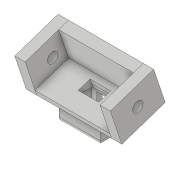
# Autodesk Inventor part: Lidar Sensor Case v2
Saved by Autodesk Inventor 2018.3 (Build 223284000, 284)
## iProperties
Created: 2019-02-04
Part Number: Lidar Sensor Case v2
Material: Generic
Document SubType Name: Modeling
Designer: aye06091
Mass: 21.1942 g
Surface Area: 105.081 cm^2
Volume: 21.1942 cm^3
Density: 1 g/cm^3
Appearance: Default
Author: aye06091
Autodesk Inventor part; units mm, degrees
ref_plane "YZ Plane" through (0, 0, 0) normal (1, 0, 0) x (0, 1, 0)
ref_plane "XZ Plane" through (0, 0, 0) normal (0, 1, 0) x (-1, 0, 0)
ref_plane "XY Plane" through (0, 0, 0) normal (0, 0, 1) x (1, 0, 0)
sketch "Sketch8" plane through (0, 0, 0) normal (1, 0, 0) x (0, 1, 0)
  line L0 (-3.8078, 7.851) -> (3.0591, -12.6251)
  line L1 (-0.2897, -12.6251) -> (-4.6863, 0.485)
  line L2 (3.0591, -12.6251) -> (-0.2897, -12.6251)
  line L3 (-4.6863, 0.485) -> (-6.818, 6.8414)
  line L4 (-3.8078, 7.851) -> (-6.818, 6.8414)
  point P0 (0, 0)
  constraints: 10 end point, 1 horizontal, 1 perpendicular
extrude "Extrusion6" add sketch "Sketch8" along normal blind 45.72
sketch "Sketch11" plane through (0, 0, 0) normal (-1, 0, 0) x (0, 0, 1)
  line L0 (0.485, -4.6863) -> (-12.6251, -0.2897) projected
  line L1 (7.851, -6.8159) -> (0.485, -6.8159) projected
  line L2 (7.851, -6.8159) -> (0.485, -6.8159)
  line L3 (0.485, -6.8159) -> (0.485, -4.6863)
  line L4 (-12.6251, -0.2897) -> (0.485, -4.6863)
  line L5 (7.851, -3.8078) -> (-12.6251, 3.0591) projected
  line L6 (0.485, -6.8159) -> (7.851, -6.8159) projected
  line L7 (13.9082, 14.2533) -> (7.851, -3.808)
  line L8 (7.851, -3.808) -> (-18.639, 5.076)
  line L9 (-18.639, 5.076) -> (-12.5817, 23.1373)
  line L10 (-12.5817, 23.1373) -> (13.9082, 14.2533)
  point P0 (0, 0)
  dimension "d73" = 27.94
  dimension "d74" = 18.54
  dimension "d76" = 0
  dimension "d88" = 19.05
  constraints: 14 end point, 2 parallel, 2 perpendicular, 1 point on line
  measures "d73" distance of L9.end L7.start
  measures "d74" angle of L6 L8
  measures "d76" distance from line of L5 L8.end
  measures "d88" distance of L8.end L9.end
extrude "Extrusion8" add sketch "Sketch11" along normal blind 6.35
sketch "Sketch13" plane through (0, -3.8078, 7.851) normal (0, 0.9481042, 0.3179598) x (1, 0, 0)
  line L0 (0, 0) -> (0, 21.5968) projected
  line L1 (16.51, 18.0408) -> (29.21, 18.0408)
  line L2 (29.21, 18.0408) -> (29.21, 10.4208)
  line L3 (29.21, 10.4208) -> (16.51, 10.4208)
  line L4 (16.51, 10.4208) -> (16.51, 18.0408)
  point P0 (0, 8.6543)
  dimension "d55" = 7.62
  dimension "d56" = 12.7
  dimension "d57" = 16.51
  constraints: 8 end point, 2 parallel, 1 horizontal, 1 perpendicular
  measures "d55" distance of L3.end L1.start
  measures "d56" distance of L2.end L3.end
  measures "d57" distance between parallel lines of L0 L4
extrude "Extrusion10" cut sketch "Sketch13" against normal blind 25.4
sketch "Sketch15" plane through (0, 0, 0) normal (1, 0, 0) x (0, 0, -1)
  line L0 (-0.485, -6.8159) -> (-7.851, -6.8159) projected
  line L1 (6.5678, 21.1205) -> (12.5883, 23.1395)
  line L2 (12.5883, 23.1395) -> (18.6455, 5.0782)
  line L3 (18.6455, 5.0782) -> (12.6251, 3.0591)
  line L4 (12.6251, 3.0591) -> (6.5678, 21.1205)
  dimension "d67" = 6.35
  dimension "d68" = 18.54
  dimension "d69" = 0
  dimension "d70" = 0
  dimension "d87" = 19.05
  constraints: 8 end point, 2 parallel, 1 perpendicular
  measures "d67" distance of L1.start L1.end
  measures "d68" angle of L0 L3
  measures "d69" distance of point (12.625, 3.059) L3.end
  measures "d70" distance of point (12.625, 3.059) L3.end
  measures "d87" distance of L3.end L1.start
extrude "Extrusion11" add sketch "Sketch15" along normal blind 45.72
sketch "Sketch17" plane through (45.72, 0, 0) normal (1, 0, 0) x (0, 0, -1)
  line L0 (-7.851, -3.808) -> (-13.9082, 14.2533) projected
  line L1 (-7.851, -3.808) -> (-13.9082, 14.2533)
  line L2 (-13.9082, 14.2533) -> (12.5883, 23.1395)
  line L3 (12.5883, 23.1395) -> (18.6456, 5.0782)
  line L4 (18.6456, 5.0782) -> (-7.851, -3.808)
  point P0 (0, 0)
  constraints: 8 end point, 2 parallel, 1 perpendicular
extrude "Extrusion12" add sketch "Sketch17" along normal blind 6.35
sketch "Sketch19" plane through (45.72, 5.0782, -18.6456) normal (0, -0.9481019, -0.3179666) x (1, 0, 0)
  line L0 (0, 6.3501) -> (0, 0.0001) projected
  line L1 (6.35, 27.947) -> (0, 27.947)
  line L2 (0, 27.947) -> (0, 0.0001)
  line L3 (0, 0.0001) -> (6.35, 0.0001)
  line L4 (6.35, 0.0001) -> (6.35, 27.947)
  line L5 (-45.72, 6.3501) -> (0, 6.3501) projected
  line L6 (0, 0.0001) -> (0, 0.0001)
  line L7 (0, 0.0001) -> (0, 6.3501)
  line L8 (0, 6.3501) -> (0, 6.3501)
  line L9 (0, 6.3501) -> (0, 0.0001)
  line L10 (-45.72, 0.007) -> (-52.07, 0.007) projected
  line L11 (-52.07, 0.007) -> (-45.72, 0.007)
  line L12 (-45.72, 0.007) -> (-45.72, 27.947)
  line L13 (-45.72, 27.947) -> (-52.07, 27.947)
  line L14 (-52.07, 27.947) -> (-52.07, 0.007)
  point P0 (-45.72, 19.2926)
  constraints: 24 end point, 6 equal length, 3 horizontal, 3 perpendicular, 1 point on line
extrude "Extrusion13" add sketch "Sketch19" along normal blind 3.175
sketch "Sketch20" plane through (0, 5.0782, -18.6455) normal (0, -0.9481019, -0.3179666) x (1, 0, 0)
  line L0 (45.72, 0) -> (0, 0)
  line L1 (0, 0) -> (0, 6.35)
  line L2 (0, 6.35) -> (45.72, 6.35)
  line L3 (45.72, 6.35) -> (45.72, 0)
  point P0 (0, 19.2926)
  constraints: 8 end point, 2 parallel, 1 horizontal, 1 perpendicular
extrude "Extrusion14" add sketch "Sketch20" along normal blind 3.175
sketch "Sketch21" plane through (0, 0, 0) normal (1, 0, 0) x (0, 0, -1)
  line L0 (19.6485, 2.0658) -> (13.6346, 0.0489) projected
  line L1 (13.6346, 0.0489) -> (12.6251, 3.0591) projected
  line L2 (12.6251, 3.0591) -> (12.6251, -0.2897) projected
  line L3 (12.6251, -0.2897) -> (-6.8414, -6.818) projected
  line L4 (-0.485, -4.6863) -> (-0.485, -4.6865) projected
  line L5 (19.6485, 2.0657) -> (-6.8414, -6.8182) projected
  line L6 (19.6485, 2.0657) -> (19.6485, 2.0658) projected
  line L7 (12.6251, 3.0591) -> (13.6346, 0.0489)
  line L8 (12.6251, -0.2897) -> (13.6346, 0.0489)
  line L9 (12.6251, 3.0591) -> (12.6251, -0.2897)
  point P0 (0, 0)
  point P1 (-6.8415, -6.8181)
  constraints: 6 end point, 2 collinear, 1 perpendicular
extrude "Extrusion15" add sketch "Sketch21" along normal blind 45.72
sketch "Sketch22" plane through (16.51, -1.0818, -10.2631) normal (0, 0.9481042, 0.3179598) x (1, 0, 0)
  line L0 (12.7, -7.62) -> (12.7, 0) projected
  line L1 (12.7, 0) -> (0, 0) projected
  line L2 (0, 0) -> (12.7, 0)
  line L3 (12.7, 0) -> (12.7, -7.62)
  line L4 (12.7, -7.62) -> (0, -7.62)
  line L5 (0, -7.62) -> (0, 0)
  point P0 (-16.51, -9.3866)
  constraints: 8 end point, 2 parallel, 1 horizontal, 1 perpendicular
extrude "Extrusion16" cut sketch "Sketch22" against normal blind 45.72
sketch "Sketch23" plane through (52.07, 0, 0) normal (1, 0, 0) x (0, 0, -1)
  circle A0 centre (2.8734, 8.1606) radius 3.175
  point P0 (0, 0)
  dimension "d89" = 6.35
  constraints: 1 centre point
  measures "d89" diameter of A0
extrude "Extrusion17" cut sketch "Sketch23" against normal blind 76.2
ref_plane "Work Plane1" through (0, -6.818, 6.8414) normal (0, -1, 0) x (1, 0, 0)
sketch "Sketch25" plane through (0, -6.818, 6.8414) normal (0, -1, 0) x (1, 0, 0)
  line L0 (35.56, -20.2796) -> (35.56, -3.5301)
  line L1 (35.56, -3.5301) -> (32.385, -3.5301)
  line L2 (32.385, -3.5301) -> (32.385, -20.2796)
  line L3 (32.385, -6.7051) -> (10.16, -6.7051)
  line L4 (10.16, -6.7051) -> (10.16, -3.5301)
  line L5 (10.16, -3.5301) -> (32.385, -3.5301)
  line L6 (32.385, -3.5301) -> (32.385, -6.7051)
  line L7 (10.16, -6.7051) -> (13.335, -6.7051)
  line L8 (13.335, -6.7051) -> (13.335, -20.2796)
  line L9 (10.16, -20.2796) -> (10.16, -6.7051)
  line L10 (13.335, -20.2796) -> (32.385, -20.2796)
  line L11 (32.385, -20.2796) -> (32.385, -23.4546)
  line L12 (32.385, -23.4546) -> (13.335, -23.4546)
  line L13 (13.335, -23.4546) -> (13.335, -20.2796)
  line L14 (29.21, -17.1046) -> (16.51, -17.1046) projected
  line L15 (29.21, -9.8801) -> (29.21, -17.1046) projected
  line L16 (16.51, -9.8801) -> (29.21, -9.8801) projected
  line L17 (16.51, -17.1046) -> (16.51, -9.8801) projected
  line L18 (32.385, -23.4546) -> (35.56, -23.4546)
  line L19 (35.56, -23.4546) -> (35.56, -3.5301)
  line L20 (35.56, -3.5301) -> (32.385, -3.5301)
  line L21 (32.385, -3.5301) -> (32.385, -23.4546)
  line L22 (32.385, -3.5301) -> (10.16, -3.5301)
  line L23 (10.16, -3.5301) -> (10.16, -6.7051)
  line L24 (10.16, -6.7051) -> (32.385, -6.7051)
  line L25 (32.385, -6.7051) -> (32.385, -3.5301)
  line L26 (10.16, -6.7051) -> (13.335, -6.7051)
  line L27 (13.335, -6.7051) -> (13.335, -23.4546)
  line L28 (13.335, -23.4546) -> (10.16, -23.4546)
  line L29 (10.16, -23.4546) -> (10.16, -6.7051)
  line L30 (32.385, -20.2796) -> (13.335, -20.2796)
  line L31 (13.335, -20.2796) -> (13.335, -23.4546)
  line L32 (13.335, -23.4546) -> (32.385, -23.4546)
  line L33 (32.385, -23.4546) -> (32.385, -20.2796)
  line L34 (35.56, -3.5301) -> (32.385, -3.5301)
  line L35 (32.385, -3.5301) -> (32.385, -23.4546)
  line L36 (32.385, -23.4546) -> (35.56, -23.4546)
  line L37 (35.56, -23.4546) -> (35.56, -3.5301)
  point P0 (0, -6.8414)
  dimension "d102" = 3.175
  dimension "d103" = 3.175
  dimension "d104" = 3.175
  dimension "d105" = 3.175
  dimension "d106" = 3.175
  dimension "d107" = 3.175
  dimension "d108" = 3.175
  dimension "d109" = 3.175
  constraints: 68 end point, 16 parallel, 8 horizontal, 8 perpendicular, 3 point on line
  measures "d102" distance between parallel lines of L12 L10
  measures "d103" distance between parallel lines of L15 L2
  measures "d104" distance between parallel lines of L3 L16
  measures "d105" distance between parallel lines of L8 L17
  measures "d106" distance between parallel lines of L14 L10
  measures "d107" distance between parallel lines of L3 L5
  measures "d108" distance between parallel lines of L2 L0
  measures "d109" distance between parallel lines of L9 L8
extrude "Extrusion18" add sketch "Sketch25" against normal blind 3.81 contours L19 L18 L11 L2 L1 L0 | L2 L3 L4 L5 | L12 L13 L10 L11 | L28 L29 L9 L3 L8 L13
sketch "Sketch26" plane through (35.56, -6.818, 3.3114) normal (1, 0, 0) x (0, 0, -1)
  line L0 (7.8311, 3.81) -> (19.9245, 3.81) projected
  line L1 (7.8311, 3.81) -> (19.9245, 3.81)
  line L2 (19.9245, 3.81) -> (19.9245, 7.8658)
  line L3 (19.9245, 7.8658) -> (7.8311, 3.81)
  point P0 (3.3114, 6.818)
  constraints: 6 end point, 1 horizontal, 1 vertical
extrude "Extrusion19" add sketch "Sketch26" against normal blind 25.4
sketch "Sketch27" plane through (16.51, -1.0818, -10.2632) normal (0, 0.9481013, 0.3179684) x (1, 0, 0)
  line L0 (0, -6.0578) -> (12.7, -6.0578)
  line L1 (12.7, -6.0578) -> (12.7, 0)
  line L2 (12.7, 0) -> (0, 0)
  line L3 (0, 0) -> (0, -6.0578)
  point P0 (-16.51, -9.3865)
  constraints: 8 end point, 2 parallel, 1 horizontal, 1 perpendicular
extrude "Extrusion20" cut sketch "Sketch27" against normal blind 25.4
sketch "Sketch28" plane through (0, -6.818, 6.8414) normal (0, -1, 0) x (1, 0, 0)
  line L0 (10.16, -3.5301) -> (10.16, -23.4546) projected
  line L1 (35.56, -23.4546) -> (35.56, -3.5301) projected
  line L2 (35.56, -3.5301) -> (10.16, -3.5301) projected
  line L3 (32.385, -6.7051) -> (13.335, -6.7051) projected
  line L4 (32.385, -6.7051) -> (32.385, -20.2796) projected
  line L5 (32.385, -20.2796) -> (13.335, -20.2796) projected
  line L6 (13.335, -20.2796) -> (13.335, -6.7051) projected
  line L7 (35.56, -23.4546) -> (29.21, -23.4546)
  line L8 (29.21, -23.4546) -> (29.21, -20.2796)
  line L9 (29.21, -20.2796) -> (35.56, -20.2796)
  line L10 (35.56, -20.2796) -> (35.56, -23.4546)
  line L11 (10.16, -23.4546) -> (16.51, -23.4546)
  line L12 (16.51, -23.4546) -> (16.51, -20.2796)
  line L13 (16.51, -20.2796) -> (10.16, -20.2796)
  line L14 (10.16, -20.2796) -> (10.16, -23.4546)
  line L15 (13.335, -6.7051) -> (13.335, -11.3612) projected
  line L16 (10.16, -20.2796) -> (13.335, -20.2796)
  line L17 (13.335, -20.2796) -> (13.335, -6.7051)
  line L18 (13.335, -6.7051) -> (10.16, -6.7051)
  line L19 (10.16, -6.7051) -> (10.16, -20.2796)
  line L20 (10.16, -3.5301) -> (35.56, -3.5301) projected
  line L21 (10.16, -6.7051) -> (35.56, -6.7051)
  line L22 (35.56, -6.7051) -> (35.56, -3.5301)
  line L23 (35.56, -3.5301) -> (10.16, -3.5301)
  line L24 (10.16, -3.5301) -> (10.16, -6.7051)
  line L25 (35.56, -6.7051) -> (32.385, -6.7051)
  line L26 (32.385, -6.7051) -> (32.385, -20.2796)
  line L27 (32.385, -20.2796) -> (35.56, -20.2796)
  line L28 (35.56, -20.2796) -> (35.56, -6.7051)
  point P0 (0, -6.8414)
  dimension "d116" = 6.35
  dimension "d117" = 6.35
  constraints: 40 end point, 10 parallel, 5 horizontal, 5 perpendicular, 2 point on line
  measures "d116" distance between parallel lines of L0 L12
  measures "d117" distance between parallel lines of L8 L1
extrude "Extrusion21" add sketch "Sketch28" along normal blind 8.255 contours L2 L1 L21 L3 L18 L0 | L18 L6 L13 L0 | L13 L5 L12 L11 L0 | L1 L9 L4 L21 | L1 L7 L8 L5 L9
sketch "Sketch29" plane through (0, -15.073, 6.8414) normal (0, -1, 0) x (1, 0, 0)
  line L0 (35.56, -23.4546) -> (35.56, -3.5301) projected
  line L1 (35.56, -3.5301) -> (10.16, -3.5301) projected
  line L2 (35.56, -6.3565) -> (35.56, -23.4546) projected
  line L3 (10.16, -23.4546) -> (35.56, -23.4546)
  line L4 (35.56, -23.4546) -> (35.56, -20.2796)
  line L5 (35.56, -20.2796) -> (10.16, -20.2796)
  line L6 (10.16, -20.2796) -> (10.16, -23.4546)
  line L7 (35.56, -3.5301) -> (35.56, -6.3565) projected
  line L8 (10.16, -23.4546) -> (10.16, -6.3565) projected
  line L9 (35.56, -3.5301) -> (10.16, -3.5301)
  line L10 (10.16, -3.5301) -> (10.16, -6.7051)
  line L11 (10.16, -6.7051) -> (35.56, -6.7051)
  line L12 (35.56, -6.7051) -> (35.56, -3.5301)
  line L13 (35.56, -6.7051) -> (32.385, -6.7051)
  line L14 (32.385, -6.7051) -> (32.385, -20.2796)
  line L15 (32.385, -20.2796) -> (35.56, -20.2796)
  line L16 (35.56, -20.2796) -> (35.56, -6.7051)
  line L17 (13.335, -6.7051) -> (10.16, -6.7051)
  line L18 (10.16, -6.7051) -> (10.16, -20.2796)
  line L19 (10.16, -20.2796) -> (13.335, -20.2796)
  line L20 (13.335, -20.2796) -> (13.335, -6.7051)
  point P0 (0, -6.8414)
  dimension "d120" = 3.175
  constraints: 32 end point, 8 parallel, 4 horizontal, 4 perpendicular, 2 point on line
  measures "d120" distance between parallel lines of L11 L1
extrude "Extrusion22" add sketch "Sketch29" along normal blind 3.175
fillet "Fillet1" radius 3.175 4 edges at (22.86, -18.248, 3.3114) (10.16, -18.248, -6.6509) (35.56, -18.248, -6.6509) (22.86, -18.248, -16.6132)
equation "\"d57\" = d58"
equation "\"d58\" = 16.51"
body "Solid3"
